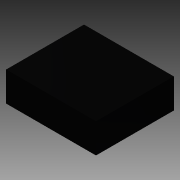
# Autodesk Inventor part: MCP130T-315I_TT
Saved by Autodesk Inventor 2015 SP1 (Build 190203100, 203)
## iProperties
Created: 2015-10-19
Part Number: MCP130T-315I_TT
Material: Generic
Document SubType Name: Modeling
Designer: Kartikye
Density: 1 g/cm^3
Appearance: SOT95P237X112-3N, MCP130T-315I_TT
Author: Kartikye
Autodesk Inventor part; units mm, degrees
ref_plane "YZ Plane" through (0, 0, 0) normal (1, 0, 0) x (0, 1, 0)
ref_plane "XZ Plane" through (0, 0, 0) normal (0, 1, 0) x (-1, 0, 0)
ref_plane "XY Plane" through (0, 0, 0) normal (0, 0, 1) x (1, 0, 0)
sketch "SOT95P237X112-3N, MCP130T-315I_TT_86" plane through (0, 0, 0) normal (0, 0, 1) x (1, 0, 0)
  line L0 (-1.524, 1.3208) -> (1.524, 1.3208)
  line L1 (1.524, 1.3208) -> (1.524, -1.3208)
  line L2 (1.524, -1.3208) -> (-1.524, -1.3208)
  line L3 (-1.524, -1.3208) -> (-1.524, 1.3208)
  constraints: 8 end point
extrude "Extrusion1" add sketch "SOT95P237X112-3N, MCP130T-315I_TT_86" along normal blind 1
body "Solid1"
